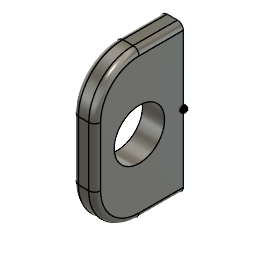
Atlas_Shelf_Corner v.1.0 (Autodesk Fusion 360 archive; units mm, degrees)
design "Atlas_ShelfTab_ST001"
part number: 2026-07-26-16-47-24-662
Autodesk Fusion 360 part; units mm, degrees
sketch "Sketch1" plane through (0, 0, 0) normal (0, 0, 1) x (1, 0, 0)
  line L0 (0.9525, 6.35) -> (-0.9525, 6.35)
  line L1 (-0.9525, 6.35) -> (-0.9525, -6.35)
  line L2 (-0.9525, -6.35) -> (0.9525, -6.35)
  line L3 (0.9525, -6.35) -> (0.9525, 6.35)
  line L4 (0.9525, 6.35) -> (-0.9525, -6.35) construction
  line L5 (-0.9525, 6.35) -> (0.9525, -6.35) construction
  dimension "d7" = 1.905
  dimension "d8" = 12.7
  constraint horizontal L0
  constraint perpendicular L0 L1
  constraint parallel L0 L2
  constraint parallel L1 L3
  constraint coincident L4 origin
  constraint coincident L5 origin
  measures "d7" distance of L1.end L2.end
  measures "d8" distance of L0.end L1.end
extrude "Extrude1" add sketch "Sketch1" along normal blind 7.62
sketch "Sketch2" plane through (0.9525, 0, 0) normal (1, 0, 0) x (0, 0, -1)
  line L0 (0, -6.35) -> (0, 6.35)
  line L1 (0, 6.35) -> (-7.62, 6.35)
  line L2 (-7.62, 6.35) -> (-7.62, -6.35)
  line L3 (-7.62, -6.35) -> (0, -6.35)
  circle A0 centre (-3.7773, 0) radius 2.159
  dimension "d11" = 4.318
  measures "d11" diameter of A0
extrude "Extrude2" cut sketch "Sketch2" against normal blind 12.7 contours A0
sketch "Sketch3" plane through (0, 0, 0) normal (0, 0, -1) x (-1, 0, 0)
  line L0 (-0.9525, 6.35) -> (-0.9525, -6.35)
  line L1 (-0.9525, -6.35) -> (0.9525, -6.35)
  line L2 (0.9525, -6.35) -> (0.9525, 6.35)
  line L3 (0.9525, 6.35) -> (-0.9525, 6.35)
  point P0 (-0.9525, 0)
  constraint midpoint L0 P0
fillet "Fillet1" radius 3.81 2 edges at (0, 6.35, 7.62) (0, -6.35, 7.62)
fillet "Fillet2" radius 0.508 10 edges at (0.9525, -6.35, 1.905) (0.9525, -5.2341, 6.5041) (0.9525, 0, 7.62) (0.9525, 5.2341, 6.5041) (0.9525, 6.35, 1.905) (-0.9525, 6.35, 1.905) (-0.9525, 5.2341, 6.5041) (-0.9525, 0, 7.62) (-0.9525, -5.2341, 6.5041) (-0.9525, -6.35, 1.905)
equation "tabHeight = 0.3 in"
equation "tabWidth = 0.5 in"
equation "tabThickness = 0.075 in"
equation "pinSize = 0.15 in"
equation "pinHoleClearance = 0.02 in"
equation "pinHoleDiameter = pinSize + pinHoleClearance"
equation "d7 = tabThickness"
equation "d8 = tabWidth"
equation "d9 = tabHeight"
equation "d11 = pinHoleDiameter"

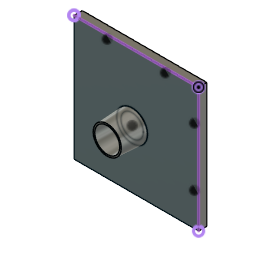
design "Atlas_Shelf_P002"
part number: 2026-07-26-17-04-48-127
Autodesk Fusion 360 part; units mm, degrees
sketch "Sketch1" plane through (0, 0, 0) normal (0, 0, 1) x (1, 0, 0)
  line L0 (19.05, -19.05) -> (-19.05, -19.05)
  line L1 (-19.05, -19.05) -> (-19.05, 19.05)
  line L2 (-19.05, 19.05) -> (19.05, 19.05)
  line L3 (19.05, 19.05) -> (19.05, -19.05)
  line L4 (19.05, -19.05) -> (-19.05, 19.05) construction
  line L5 (-19.05, -19.05) -> (19.05, 19.05) construction
  dimension "d9" = 38.1
  dimension "d10" = 38.1
  constraint horizontal L0
  constraint perpendicular L0 L1
  constraint parallel L0 L2
  constraint parallel L1 L3
  constraint coincident L4 origin
  constraint coincident L5 origin
  measures "d9" distance of L1.end L2.end
  measures "d10" distance of L0.end L1.end
extrude "Extrude1" add sketch "Sketch1" along normal blind 2.54
sketch "Sketch2" plane through (0, 0, 2.54) normal (0, 0, 1) x (1, 0, 0)
  line L0 (19.05, 19.05) -> (-19.05, 19.05)
  line L1 (-19.05, 19.05) -> (-19.05, -19.05)
  line L2 (-19.05, -19.05) -> (19.05, -19.05)
  line L3 (19.05, -19.05) -> (19.05, 19.05)
  line L4 (19.05, 19.05) -> (-19.05, 19.05)
  line L5 (19.05, -19.05) -> (19.05, 19.05)
  line L6 (-19.05, 19.05) -> (19.05, 19.05)
  line L7 (19.05, 19.05) -> (19.05, -19.05)
  circle A0 centre (-1.27, -1.27) radius 4.699
  circle A1 centre (-1.27, -1.27) radius 3.429
  point P0 (17.78, 8.89)
  point P1 (17.78, -8.89)
  dimension "d13" = 10.16
  dimension "d14" = 1.27
  dimension "d15" = 27.94
  dimension "d16" = 1.27
  dimension "d49" = 9.398
  dimension "d50" = 20.32
  dimension "d51" = 20.32
  dimension "d54" = 6.858
  constraint concentric A0 A1
  measures "d13" distance of P0 L4
  measures "d14" distance of P0 L5
  measures "d15" distance of L4 P1
  measures "d16" distance of L5 P1
  measures "d49" diameter of A0
  measures "d50" distance of L0 A0.centre
  measures "d51" distance of L5 A0.centre
  measures "d54" diameter of A1
sketch "Sketch3" plane through (0, 0, 2.54) normal (0, 0, 1) x (1, 0, 0)
  line L0 (19.05, 19.05) -> (-19.05, 19.05)
  line L1 (19.05, -19.05) -> (19.05, 19.05)
  line L2 (19.05, 19.05) -> (-19.05, 19.05)
  point P0 (8.89, 17.78)
  point P1 (-8.89, 17.78)
  dimension "d27" = 1.27
  dimension "d28" = 10.16
  dimension "d29" = 1.27
  dimension "d30" = 27.94
  measures "d27" distance of P0 L0
  measures "d28" distance of P0 L1
  measures "d29" distance of P1 L2
  measures "d30" distance of L1 P1
sketch "Sketch5" plane through (0, 0, 2.54) normal (0, 0, 1) x (1, 0, 0)
extrude "Extrude3" add sketch "Sketch2" along normal blind 7.62 draft -3 contours A0
sketch "Sketch6" plane through (0, 0, 2.54) normal (0, 0, 1) x (1, 0, 0)
  circle A0 centre (-1.27, -1.27) radius 3.175
  point P0 (-1.27, -1.27)
  dimension "d59" = 6.35
  constraint coincident P0 A0.centre
  measures "d59" diameter of A0
extrude "Extrude4" cut sketch "Sketch6" against normal blind 2.54
extrude "Extrude2" [suppressed]
fillet "Fillet1" [suppressed]
equation "shelfThickness = 0.1 in"
equation "shelfWidth = 1.5 in"
equation "shelfDepth = 1.5 in"
equation "trussThickness = 0.1 in"
equation "tabInset = trussThickness / 2"
equation "tabWidth = 0.5 in"
equation "tab1Offset = tabBaseOffset + tabWidth / 2"
equation "tab2Offset = tabBaseOffset + ( tabWidth / 2 ) + tabSeparation"
equation "d9 = shelfWidth"
equation "d10 = shelfDepth"
equation "d11 = shelfThickness"
equation "d13 = tab1Offset"
equation "d14 = tabInset"
equation "d15 = tab2Offset"
equation "d16 = tabInset"
equation "tabBaseOffset = 0.15 in"
equation "tabSeparation = tabWidth + 0.2 in"
equation "d27 = tabInset"
equation "d28 = tab1Offset"
equation "d29 = tabInset"
equation "d30 = tab2Offset"
equation "columnWallThickness = 0.05 in"
equation "columnClearance = 0.25 in"
equation "bossCenterOffset = 0.5 in + columnWallThickness + columnClearance"
equation "bossDiameter = 0.37 in"
equation "bossHeight = 0.3 in"
equation "d49 = bossDiameter"
equation "d50 = bossCenterOffset"
equation "d51 = bossCenterOffset"
equation "bossWallThickness = 0.05 in"
equation "bossInnerDiameter = bossDiameter - 2 * ( bossWallThickness )"
equation "d54 = bossInnerDiameter"
equation "bossTaper = -3"
equation "d56 = bossHeight"
equation "pinDiameter = 0.25 in"
equation "d59 = pinDiameter"
